Autodesk Inventor part; units mm, degrees
(part 2 of 2)
sketch "スケッチ7" plane through (0, 0, 0) normal (0, 0, 1) x (1, 0, 0)
  line L0 (-15.4359, 10.7396) -> (-13.9558, 2.1157) projected
  line L1 (-1.1431, 4.3146) -> (-2.6232, 12.9386) projected
  line L2 (-2.6232, 12.9386) -> (-15.4359, 10.7396) projected
  line L3 (-8.5367, 11.9237) -> (-3.6088, 12.7694) projected
  line L4 (-14.4503, 10.9088) -> (-9.5223, 11.7545) projected
  line L5 (-15.4359, 10.7396) -> (-13.9558, 2.1157) projected
  line L6 (-2.6232, 12.9386) -> (-15.4359, 10.7396) projected
  line L7 (-1.1431, 4.3146) -> (-2.6232, 12.9386) projected
  line L8 (-8.0423, 3.1306) -> (-12.9702, 2.2848) projected
  line L9 (-13.9558, 2.1157) -> (-1.1431, 4.3146) projected
  line L10 (-13.9558, 2.1157) -> (-1.1431, 4.3146) projected
  line L11 (-7.0686, 4.7383) -> (-2.1618, 5.6993) projected
  line L12 (-1.1804, 5.8915) -> (-7.5593, 4.6422) projected
  line L13 (-7.5593, 4.6422) -> (-1.1804, 5.8915) projected
  line L14 (-9.0295, 11.8391) -> (-7.5495, 3.2152) projected
  line L15 (-7.5495, 3.2152) -> (-9.0295, 11.8391) projected
  line L16 (15.4359, 10.7396) -> (13.9558, 2.1157) projected
  line L17 (1.1431, 4.3146) -> (2.6232, 12.9386) projected
  line L18 (2.6232, 12.9386) -> (15.4359, 10.7396) projected
  line L19 (3.6088, 12.7694) -> (8.5367, 11.9237) projected
  line L20 (9.5223, 11.7545) -> (14.4503, 10.9088) projected
  line L21 (15.4359, 10.7396) -> (13.9558, 2.1157) projected
  line L22 (2.6232, 12.9386) -> (15.4359, 10.7396) projected
  line L23 (1.1431, 4.3146) -> (2.6232, 12.9386) projected
  line L24 (2.1618, 5.6993) -> (7.0686, 4.7383) projected
  line L25 (7.5593, 4.6422) -> (1.1804, 5.8915) projected
  line L26 (1.1804, 5.8915) -> (7.5593, 4.6422) projected
  line L27 (7.5495, 3.2152) -> (9.0295, 11.8391) projected
  line L28 (9.0295, 11.8391) -> (7.5495, 3.2152) projected
  line L29 (13.9558, 2.1157) -> (1.1431, 4.3146) projected
  line L30 (13.9558, 2.1157) -> (1.1431, 4.3146) projected
  line L31 (12.9702, 2.2848) -> (8.0423, 3.1306) projected
  line L32 (-291.6857, -36.6711) -> (324.2647, 69.0399) projected
  line L33 (-324.2647, 69.0399) -> (291.6857, -36.6711) projected
  line L34 (0, 0) -> (0, 10) construction
  line L35 (0, 0) -> (10, 0) construction
  line L36 (0, 0) -> (10, 0) construction
  line L37 (-18, 1.5) -> (-17, 1.5) construction
  line L38 (-18, 11.5) -> (-18, -11.5) construction
  line L39 (-18, -11.5) -> (-20, -11.5) construction
  line L40 (-20, -11.5) -> (-20, 11.5) construction
  line L41 (-28.75, 11.5) -> (-28.75, -11.5) construction
  line L42 (-28.75, -11.5) -> (-20, -11.5) construction
  line L43 (-17, -1.5) -> (-18, -1.5) construction
  line L44 (0, 0) -> (0, 10) construction
  line L45 (17, -20) -> (-17, -20) construction
  line L46 (-20, 11.5) -> (-18, 11.5) construction
  line L47 (-20, 11.5) -> (-28.75, 11.5) construction
  line L48 (-10.5, 21) -> (-14.5, 21) construction
  circle A0 centre (-12.5, 23.5) radius 1 construction
  line L49 (-14.5, 26) -> (-10.5, 21) construction
  line L50 (-10.5, 26) -> (-14.5, 21) construction
  line L51 (-10.5, 26) -> (-10.5, 21) construction
  line L52 (10.5, 26) -> (10.5, 21) construction
  circle A1 centre (12.5, 23.5) radius 1 construction
  line L53 (10.5, 21) -> (14.5, 21) construction
  line L54 (10.5, 26) -> (14.5, 21) construction
  line L55 (10.5, 21) -> (14.5, 26) construction
  circle A2 centre (0, 0) radius 16 construction
  circle A3 centre (0, 0) radius 7.5 construction
  line L56 (20, 11.5) -> (28.75, 11.5) construction
  line L57 (28.75, 11.5) -> (28.75, -11.5) construction
  line L58 (-17, -20) -> (-17, 26) construction
  line L59 (-14.5, 26) -> (-14.5, -20) construction
  line L60 (-17, 26) -> (17, 26) construction
  line L61 (17, -1.5) -> (18, -1.5) construction
  line L62 (18, 1.5) -> (17, 1.5) construction
  line L63 (18, 11.5) -> (18, -11.5) construction
  line L64 (20, 11.5) -> (18, 11.5) construction
  line L65 (18, -11.5) -> (20, -11.5) construction
  line L66 (20, -11.5) -> (20, 11.5) construction
  line L67 (28.75, -11.5) -> (20, -11.5) construction
  line L68 (14.5, 26) -> (14.5, -20) construction
  line L69 (17, 26) -> (17, -20) construction
  line L70 (-14.5, -15) -> (-10.5, -15) construction
  circle A4 centre (-12.5, -17.5) radius 1 construction
  line L71 (-14.5, -15) -> (-10.5, -20) construction
  line L72 (-10.5, -15) -> (-14.5, -20) construction
  line L73 (-10.5, -15) -> (-10.5, -20) construction
  line L74 (10.5, -15) -> (14.5, -15) construction
  circle A5 centre (12.5, -17.5) radius 1 construction
  line L75 (10.5, -20) -> (10.5, -15) construction
  line L76 (14.5, -15) -> (10.5, -20) construction
  line L77 (10.5, -15) -> (14.5, -20) construction
  line L78 (29.25, -41.1836) -> (-29.25, -41.1836) construction
  line L79 (-29.25, -41.1836) -> (29.25, -41.1836) projected
  line L80 (0, 0) -> (0, 10) construction
  line L81 (0, 0) -> (0, 10) construction
  line L82 (20, 11.5) -> (18, 11.5) construction
  line L83 (2.6232, 12.9386) -> (1.1431, 4.3146) construction
  line L84 (9.0295, 11.8391) -> (2.6232, 12.9386) construction
  line L85 (8.4099, 11.1845) -> (3.4819, 12.0302) construction
  line L86 (3.4819, 12.0302) -> (2.6362, 7.1023) construction
  line L87 (8.4099, 11.1845) -> (2.6362, 7.1023) construction
  line L88 (7.5641, 6.2565) -> (3.4819, 12.0302) construction
  line L89 (2.6362, 7.1023) -> (7.5641, 6.2565) construction
  line L90 (7.9301, 5.4327) -> (1.5237, 6.5322) construction
  line L91 (7.5641, 6.2565) -> (8.4099, 11.1845) construction
  line L92 (13.4777, 5.2416) -> (14.3234, 10.1696) construction
  line L93 (17, 8.5) -> (17, -8.5) construction
  line L94 (7.5495, 3.2152) -> (9.0295, 11.8391) construction
  line L95 (9.3955, 11.0153) -> (8.5497, 6.0874) construction
  line L96 (8.5497, 6.0874) -> (13.4777, 5.2416) construction
  line L97 (13.4777, 5.2416) -> (9.3955, 11.0153) construction
  line L98 (13.9005, 7.7056) -> (8.9726, 8.5513) construction
  line L99 (14.3234, 10.1696) -> (9.3955, 11.0153) construction
  line L100 (15.4359, 10.7396) -> (9.0295, 11.8391) construction
  line L101 (14.1851, 3.4517) -> (7.8081, 4.722) construction
  line L102 (10.5062, 2.7077) -> (11.0137, 5.6645) construction
  line L103 (13.9558, 2.1157) -> (15.4359, 10.7396) construction
  line L104 (7.5495, 3.2152) -> (13.9558, 2.1157) construction
  line L105 (9.0295, 11.8391) -> (7.5495, 3.2152) construction
  circle A6 centre (0, 0) radius 4.25 construction
  line L106 (1.1431, 4.3146) -> (7.5495, 3.2152) construction
  line L107 (29.25, 8.5) -> (17, 8.5) construction
  line L108 (-2.6232, 12.9386) -> (-1.1431, 4.3146) construction
  line L109 (-3.4819, 12.0302) -> (-2.6362, 7.1023) construction
  line L110 (-8.4099, 11.1845) -> (-3.4819, 12.0302) construction
  line L111 (-7.5641, 6.2565) -> (-3.4819, 12.0302) construction
  line L112 (-8.4099, 11.1845) -> (-2.6362, 7.1023) construction
  line L113 (-7.987, 8.7205) -> (-3.059, 9.5662) construction
  line L114 (-4.5927, 3.7226) -> (-5.1001, 6.6794) construction
  line L115 (-2.6362, 7.1023) -> (-7.5641, 6.2565) construction
  line L116 (-7.9301, 5.4327) -> (-1.5237, 6.5322) construction
  line L117 (-1.1431, 4.3146) -> (-7.5495, 3.2152) construction
  line L118 (-13.4777, 5.2416) -> (-9.3955, 11.0153) construction
  line L119 (-10.5062, 2.7077) -> (-11.0137, 5.6645) construction
  line L120 (-8.5497, 6.0874) -> (-13.4777, 5.2416) construction
  circle A7 centre (12.5, -17.5) radius 1 construction
  line L121 (14.5, -15) -> (10.5, -20) construction
  line L122 (10.3558, 32.528) -> (9.7395, 39.5722) construction
  line L123 (10.2875, 31.2799) -> (5.3082, 35.458) construction
  line L124 (10.3558, 32.528) -> (6.5255, 35.7419) construction
  line L125 (6.5255, 35.7419) -> (9.7395, 39.5722) construction
  line L126 (13.5697, 36.3582) -> (10.3558, 32.528) construction
  line L127 (6.5255, 35.7419) -> (13.5697, 36.3582) construction
  circle A8 centre (6.8337, 32.2199) radius 0.625 construction
  circle A9 centre (6.8337, 32.2199) radius 0.8 projected
  line L128 (9.7395, 39.5722) -> (13.5697, 36.3582) construction
  line L129 (5.3082, 35.458) -> (14.787, 36.6422) construction
  line L130 (14.787, 36.6422) -> (10.2875, 31.2799) construction
  circle A10 centre (13.6863, 32.9968) radius 1.5 construction
  circle A11 centre (13.6863, 32.9968) radius 0.8 projected
  line L131 (-17, 8.5) -> (-17, -8.5) construction
  line L132 (-7.5641, 6.2565) -> (-8.4099, 11.1845) construction
  line L133 (-7.5495, 3.2152) -> (-9.0295, 11.8391) construction
  line L134 (-14.3364, 4.3333) -> (-7.9301, 5.4327) construction
  line L135 (-7.5495, 3.2152) -> (-13.9558, 2.1157) construction
  line L136 (-13.4777, 5.2416) -> (-14.3234, 10.1696) construction
  line L137 (-15.4359, 10.7396) -> (-13.9558, 2.1157) construction
  line L138 (-13.9558, 2.1157) -> (-15.4359, 10.7396) construction
  line L139 (-14.3234, 10.1696) -> (-8.5497, 6.0874) construction
  line L140 (-13.9005, 7.7056) -> (-8.9726, 8.5513) construction
  line L141 (-14.3234, 10.1696) -> (-9.3955, 11.0153) construction
  line L142 (-15.4359, 10.7396) -> (-9.0295, 11.8391) construction
  line L143 (-9.7365, 26) -> (-17, 26) projected
  line L144 (-20, 11.5) -> (-18, 11.5) construction
  line L145 (-18, -11.5) -> (-20, -11.5) construction
  line L146 (-18, 11.5) -> (-18, -11.5) construction
  line L147 (-20, -11.5) -> (-20, 11.5) construction
  line L148 (-10.5, 26) -> (-10.5, 21) construction
  line L149 (-10.5, 21) -> (-14.5, 21) construction
  circle A12 centre (-6.8337, 32.2199) radius 0.625 construction
  circle A13 centre (-6.8337, 32.2199) radius 0.8 construction
  circle A14 centre (-6.8337, 32.2199) radius 1.5 construction
  line L150 (-5.3082, 35.458) -> (-10.2875, 31.2799) construction
  line L151 (-6.5255, 35.7419) -> (-10.3558, 32.528) construction
  line L152 (-13.5697, 36.3582) -> (-6.5255, 35.7419) construction
  line L153 (-10.0476, 36.0501) -> (-6.8337, 32.2199) construction
  line L154 (3.695, 18.0905) -> (-3.695, 18.0905) projected
  line L155 (-9.7365, 22.9366) -> (-3.695, 18.0905) projected
  circle A15 centre (-12.5, 23.5) radius 1 construction
  line L156 (-14.5, 26) -> (-10.5, 21) construction
  line L157 (-10.5, 26) -> (-14.5, 21) construction
  line L158 (-5.3082, 35.458) -> (-14.787, 36.6422) construction
  line L159 (-29.25, 8.5) -> (-17, 8.5) construction
  line L160 (-28.75, -11.5) -> (-20, -11.5) construction
  line L161 (-28.75, 11.5) -> (-28.75, -11.5) construction
  line L162 (-20, 11.5) -> (-28.75, 11.5) construction
  line L163 (-25.25, 15.774) -> (-13.111, 37.7059) projected
  line L164 (-6.6466, -20.8804) -> (-17, -20.8804) projected
  line L165 (-17, -20.8804) -> (-17, -14.5) projected
  line L166 (-25.25, -19.2406) -> (-7.307, -37.1836) projected
  line L167 (-29.25, -20.8975) -> (-8.9639, -41.1836) projected
  line L168 (-17, -14.5) -> (-25.25, -14.5) projected
  line L169 (-25.25, -14.5) -> (-25.25, -19.2406) projected
  line L170 (-7.307, -37.1836) -> (7.307, -37.1836) projected
  line L171 (-9.7395, 39.5722) -> (-6.5255, 35.7419) construction
  line L172 (-9.8077, 40.8203) -> (-5.3082, 35.458) construction
  circle A16 centre (6.8337, 32.2199) radius 1.5 construction
  line L173 (-13.111, 37.7059) -> (13.111, 37.7059) projected
  line L174 (-29.25, 41.8164) -> (29.25, 41.8164) projected
  line L175 (5.3082, 35.458) -> (9.8077, 40.8203) construction
  line L176 (9.8077, 40.8203) -> (10.2875, 31.2799) construction
  line L177 (10.2875, 31.2799) -> (12.5856, 29.3515) construction
  line L178 (9.8077, 40.8203) -> (14.787, 36.6422) construction
  line L179 (17.0851, 34.7138) -> (14.787, 36.6422) construction
  line L180 (12.5856, 29.3515) -> (17.0851, 34.7138) construction
  line L181 (-14.787, 36.6422) -> (-9.8077, 40.8203) construction
  line L182 (-13.5697, 36.3582) -> (-9.7395, 39.5722) construction
  line L183 (-14.787, 36.6422) -> (-17.0851, 34.7138) construction
  line L184 (-9.7395, 39.5722) -> (-10.3558, 32.528) construction
  line L185 (-10.3558, 32.528) -> (-13.5697, 36.3582) construction
  line L186 (-9.8077, 40.8203) -> (-10.2875, 31.2799) construction
  line L187 (-10.2875, 31.2799) -> (-14.787, 36.6422) construction
  line L188 (-17.0851, 34.7138) -> (-12.5856, 29.3515) construction
  line L189 (-12.5856, 29.3515) -> (-10.2875, 31.2799) construction
  line L190 (-9.7365, 22.9366) -> (-9.7365, 26) projected
  circle A17 centre (-13.6863, 32.9968) radius 0.625 construction
  circle A18 centre (-13.6863, 32.9968) radius 0.8 construction
  circle A19 centre (-13.6863, 32.9968) radius 1.5 construction
  line L191 (4.5158, -27.0126) -> (-4.5158, -27.0126) projected
  line L192 (29.25, -20.8975) -> (8.9639, -41.1836) projected
  line L193 (6.6466, -20.8804) -> (4.5158, -27.0126) projected
  line L194 (17, -20.8804) -> (6.6466, -20.8804) projected
  line L195 (7.307, -37.1836) -> (25.25, -19.2406) projected
  line L196 (-10.5, -15) -> (-10.5, -20) construction
  line L197 (10.5, -20) -> (10.5, -15) construction
  line L198 (10.5, -15) -> (14.5, -15) construction
  line L199 (10.5, -15) -> (14.5, -20) construction
  line L200 (17, -14.5) -> (17, -20.8804) projected
  line L201 (25.25, -14.5) -> (17, -14.5) projected
  line L202 (28.75, -11.5) -> (20, -11.5) construction
  line L203 (-17, -8.5) -> (-29.25, -8.5) construction
  line L204 (-17, -1.5) -> (-18, -1.5) construction
  line L205 (0, 0) -> (10, 0) construction
  line L206 (-18, 1.5) -> (-17, 1.5) construction
  line L207 (-29.25, -41.1836) -> (-29.25, 41.8164) construction
  line L208 (29.25, 41.8164) -> (29.25, -41.1836) construction
  line L209 (20, 11.5) -> (28.75, 11.5) construction
  line L210 (28.75, 11.5) -> (28.75, -11.5) construction
  line L211 (17, 26) -> (17, -20) construction
  line L212 (14.5, 26) -> (14.5, -20) construction
  line L213 (-4.5158, -27.0126) -> (-6.6466, -20.8804) projected
  line L214 (0, 0) -> (10, 0) construction
  circle A20 centre (0, 0) radius 7.5 construction
  circle A21 centre (0, 0) radius 16 construction
  line L215 (-14.5, 26) -> (-14.5, -20) construction
  line L216 (-9.0295, 11.8391) -> (-2.6232, 12.9386) construction
  line L217 (-14.5, -15) -> (-10.5, -15) construction
  circle A22 centre (-12.5, -17.5) radius 1 construction
  line L218 (17, -20) -> (-17, -20) construction
  line L219 (-17, -20) -> (-17, 26) construction
  line L220 (-10.5, -15) -> (-14.5, -20) construction
  line L221 (-14.5, -15) -> (-10.5, -20) construction
  line L222 (10.5, 21) -> (14.5, 21) construction
  circle A23 centre (12.5, 23.5) radius 1 construction
  line L223 (10.5, 26) -> (14.5, 21) construction
  line L224 (10.5, 21) -> (14.5, 26) construction
  line L225 (10.5, 26) -> (10.5, 21) construction
  line L226 (9.7365, 22.9366) -> (3.695, 18.0905) projected
  line L227 (9.7365, 22.9366) -> (9.7365, 26) projected
  circle A24 centre (13.6863, 32.9968) radius 0.625 construction
  line L228 (9.7365, 26) -> (17, 26) projected
  line L229 (17, 26) -> (17, 14.5) projected
  line L230 (13.111, 37.7059) -> (25.25, 15.774) projected
  line L231 (29.25, 15.7886) -> (14.2228, 41.8164) projected
  line L232 (25.25, 15.774) -> (25.25, 14.5) projected
  line L233 (25.25, 14.5) -> (17, 14.5) projected
  line L234 (17, -1.5) -> (18, -1.5) construction
  line L235 (18, -11.5) -> (20, -11.5) construction
  line L236 (18, 11.5) -> (18, -11.5) construction
  line L237 (17, -8.5) -> (29.25, -8.5) construction
  line L238 (20, -11.5) -> (20, 11.5) construction
  line L239 (-17, 26) -> (17, 26) construction
  line L240 (-25.25, 14.5) -> (-25.25, 15.774) projected
  line L241 (-17, 14.5) -> (-25.25, 14.5) projected
  line L242 (-17, 26) -> (-17, 14.5) projected
  line L243 (-29.25, 15.7886) -> (-14.2228, 41.8164) projected
  line L244 (-9.3955, 11.0153) -> (-8.5497, 6.0874) construction
  line L245 (-9.0295, 11.8391) -> (-7.5495, 3.2152) construction
  line L246 (14.3234, 10.1696) -> (8.5497, 6.0874) construction
  line L247 (18, 1.5) -> (17, 1.5) construction
  line L248 (25.25, -19.2406) -> (25.25, -14.5) projected
  line L249 (0, 0) -> (0, 10) construction
  line L250 (0, 0) -> (0, 10) construction
  line L251 (-2.6362, 7.1023) -> (-7.5641, 6.2565) construction
  line L252 (-7.987, 8.7205) -> (-3.059, 9.5662) construction
  line L253 (-8.4099, 11.1845) -> (-2.6362, 7.1023) construction
  line L254 (-7.5641, 6.2565) -> (-3.4819, 12.0302) construction
  line L255 (0, 0) -> (10, 0) construction
  line L256 (0, 0) -> (10, 0) construction
  circle A25 centre (0, 0) radius 7.5 construction
  line L257 (-18, 11.5) -> (-18, -11.5) construction
  line L258 (-18, 11.5) -> (-18, -11.5) construction
  line L259 (-14.5, -15) -> (-10.5, -15) construction
  line L260 (10.5, -15) -> (14.5, -15) construction
  line L261 (10.5, -20) -> (10.5, -15) construction
  line L262 (10.5, -15) -> (14.5, -20) construction
  line L263 (17, -20) -> (-17, -20) construction
  line L264 (17, -20) -> (-17, -20) construction
  circle A26 centre (0, 0) radius 16 construction
  circle A27 centre (0, 0) radius 16 construction
  line L265 (-10.5, -15) -> (-10.5, -20) construction
  line L266 (-10.5, -15) -> (-14.5, -20) construction
  line L267 (-14.5, 26) -> (-14.5, -20) construction
  line L268 (-14.5, 26) -> (-14.5, -20) construction
  line L269 (-17, -20) -> (-17, 26) construction
  line L270 (-17, -20) -> (-17, 26) construction
  line L271 (-10.5, 21) -> (-14.5, 21) construction
  line L272 (-7.5641, 6.2565) -> (-8.4099, 11.1845) construction
  line L273 (-17, -1.5) -> (-18, -1.5) construction
  line L274 (-10.5, 26) -> (-14.5, 21) construction
  line L275 (-14.5, 26) -> (-10.5, 21) construction
  line L276 (-10.5, 21) -> (-14.5, 21) construction
  line L277 (-10.5, 26) -> (-10.5, 21) construction
  line L278 (10.5, 21) -> (14.5, 21) construction
  line L279 (10.5, 26) -> (14.5, 21) construction
  line L280 (-9.0295, 11.8391) -> (-2.6232, 12.9386) projected
  line L281 (-18, -11.5) -> (-20, -11.5) construction
  line L282 (-18, -11.5) -> (-20, -11.5) construction
  line L283 (-18, 1.5) -> (-17, 1.5) construction
  line L284 (-18, 1.5) -> (-17, 1.5) construction
  circle A28 centre (-12.5, 23.5) radius 1 construction
  line L285 (10.5, 26) -> (10.5, 21) construction
  circle A29 centre (12.5, 23.5) radius 1 construction
  circle A30 centre (-12.5, 23.5) radius 1 construction
  line L286 (-14.5, 26) -> (-10.5, 21) construction
  line L287 (-10.5, 26) -> (-14.5, 21) construction
  circle A31 centre (-13.6863, 32.9968) radius 1.5 construction
  line L288 (-17.0851, 34.7138) -> (-12.5856, 29.3515) construction
  circle A32 centre (-6.8337, 32.2199) radius 1.5 construction
  line L289 (-10.2875, 31.2799) -> (-14.787, 36.6422) construction
  line L290 (-5.3082, 35.458) -> (-14.787, 36.6422) construction
  line L291 (-13.5697, 36.3582) -> (-9.7395, 39.5722) construction
  line L292 (-14.787, 36.6422) -> (-9.8077, 40.8203) construction
  line L293 (10.5, 21) -> (14.5, 26) construction
  line L294 (12.5856, 29.3515) -> (17.0851, 34.7138) construction
  line L295 (-14.787, 36.6422) -> (-17.0851, 34.7138) construction
  circle A33 centre (12.5, -17.5) radius 1 construction
  line L296 (14.5, -15) -> (10.5, -20) construction
  circle A34 centre (-12.5, -17.5) radius 1 construction
  line L297 (-14.5, -15) -> (-10.5, -20) construction
  circle A35 centre (-12.5, -17.5) radius 1 construction
  line L298 (-14.5, -15) -> (-10.5, -20) construction
  line L299 (-10.5, 26) -> (-10.5, 21) construction
  line L300 (-15.4359, 10.7396) -> (-9.0295, 11.8391) projected
  line L301 (-14.3364, 4.3333) -> (-7.9301, 5.4327) projected
  line L302 (-13.9558, 2.1157) -> (-15.4359, 10.7396) projected
  line L303 (-7.5495, 3.2152) -> (-13.9558, 2.1157) projected
  line L304 (-2.6232, 12.9386) -> (-1.1431, 4.3146) projected
  line L305 (0, 0) -> (0, 10) construction
  line L306 (0, 0) -> (0, 10) construction
  line L307 (-4.5927, 3.7226) -> (-5.1001, 6.6794) construction
  circle A36 centre (0, 0) radius 7.5 construction
  line L308 (0, 0) -> (10, 0) construction
  line L309 (0, 0) -> (10, 0) construction
  line L310 (10.3558, 32.528) -> (9.7395, 39.5722) construction
  line L311 (-20, 11.5) -> (-18, 11.5) construction
  line L312 (-20, 11.5) -> (-18, 11.5) construction
  line L313 (-20, -11.5) -> (-20, 11.5) construction
  line L314 (-20, 11.5) -> (-28.75, 11.5) construction
  line L315 (-28.75, 11.5) -> (-28.75, -11.5) construction
  line L316 (-28.75, -11.5) -> (-20, -11.5) construction
  line L317 (-7.9301, 5.4327) -> (-1.5237, 6.5322) projected
  line L318 (-1.1431, 4.3146) -> (-7.5495, 3.2152) projected
  line L319 (-7.5495, 3.2152) -> (-9.0295, 11.8391) projected
  line L320 (10.5, -15) -> (14.5, -15) construction
  line L321 (-20, 11.5) -> (-28.75, 11.5) construction
  line L322 (-17, -1.5) -> (-18, -1.5) construction
  line L323 (-29.25, 8.5) -> (-17, 8.5) construction
  line L324 (-28.75, 11.5) -> (-28.75, -11.5) construction
  line L325 (-28.75, -11.5) -> (-20, -11.5) construction
  line L326 (-20, -11.5) -> (-20, 11.5) construction
  line L327 (18, 11.5) -> (18, -11.5) construction
  line L328 (20, -11.5) -> (20, 11.5) construction
  line L329 (17, -1.5) -> (18, -1.5) construction
  line L330 (18, 1.5) -> (17, 1.5) construction
  line L331 (20, 11.5) -> (18, 11.5) construction
  line L332 (18, -11.5) -> (20, -11.5) construction
  line L333 (17.0851, 34.7138) -> (14.787, 36.6422) construction
  line L334 (13.5697, 36.3582) -> (10.3558, 32.528) construction
  line L335 (14.787, 36.6422) -> (10.2875, 31.2799) construction
  line L336 (10.5, 21) -> (14.5, 21) construction
  circle A37 centre (12.5, 23.5) radius 1 construction
  line L337 (10.5, 26) -> (14.5, 21) construction
  line L338 (10.5, 26) -> (10.5, 21) construction
  line L339 (10.5, 21) -> (14.5, 26) construction
  circle A38 centre (13.6863, 32.9968) radius 0.625 construction
  circle A39 centre (13.6863, 32.9968) radius 1.5 construction
  line L340 (9.8077, 40.8203) -> (14.787, 36.6422) construction
  line L341 (20, -11.5) -> (20, 11.5) construction
  line L342 (9.8077, 40.8203) -> (10.2875, 31.2799) construction
  line L343 (20, 11.5) -> (18, 11.5) construction
  line L344 (18, 1.5) -> (17, 1.5) construction
  line L345 (17, -1.5) -> (18, -1.5) construction
  line L346 (18, -11.5) -> (20, -11.5) construction
  line L347 (18, 11.5) -> (18, -11.5) construction
  line L348 (-17, 8.5) -> (-17, -8.5) construction
  line L349 (10.5, -20) -> (10.5, -15) construction
  line L350 (-17, -8.5) -> (-29.25, -8.5) construction
  line L351 (-10.5, -15) -> (-10.5, -20) construction
  line L352 (14.5, 26) -> (14.5, -20) construction
  line L353 (17, 26) -> (17, -20) construction
  line L354 (20, 11.5) -> (28.75, 11.5) construction
  line L355 (28.75, 11.5) -> (28.75, -11.5) construction
  line L356 (28.75, -11.5) -> (20, -11.5) construction
  line L357 (-8.4099, 11.1845) -> (-3.4819, 12.0302) construction
  line L358 (-3.4819, 12.0302) -> (-2.6362, 7.1023) construction
  line L359 (17, 8.5) -> (17, -8.5) construction
  line L360 (14.5, 26) -> (14.5, -20) construction
  line L361 (17, 26) -> (17, -20) construction
  line L362 (28.75, 11.5) -> (28.75, -11.5) construction
  line L363 (28.75, -11.5) -> (20, -11.5) construction
  circle A40 centre (12.5, -17.5) radius 1 construction
  line L364 (10.5, -15) -> (14.5, -20) construction
  line L365 (14.5, -15) -> (10.5, -20) construction
  line L366 (-14.5, -15) -> (-10.5, -15) construction
  line L367 (-10.5, -15) -> (-14.5, -20) construction
  line L368 (29.25, 8.5) -> (17, 8.5) construction
  line L369 (17, -8.5) -> (29.25, -8.5) construction
  line L370 (20, 11.5) -> (28.75, 11.5) construction
  line L371 (6.5255, 35.7419) -> (9.7395, 39.5722) construction
  line L372 (29.25, -41.1836) -> (-29.25, -41.1836) construction
  line L373 (5.3082, 35.458) -> (9.8077, 40.8203) construction
  line L374 (9.7395, 39.5722) -> (13.5697, 36.3582) construction
  line L375 (-9.7395, 39.5722) -> (-6.5255, 35.7419) construction
  line L376 (-9.8077, 40.8203) -> (-5.3082, 35.458) construction
  line L377 (-6.5255, 35.7419) -> (-10.3558, 32.528) construction
  line L378 (-5.3082, 35.458) -> (-10.2875, 31.2799) construction
  circle A41 centre (-6.8337, 32.2199) radius 0.625 construction
  line L379 (-9.7395, 39.5722) -> (-10.3558, 32.528) construction
  line L380 (-9.8077, 40.8203) -> (-10.2875, 31.2799) construction
  line L381 (-29.25, -41.1836) -> (-29.25, 41.8164) construction
  circle A42 centre (13.6863, 32.9968) radius 0.8 projected
  line L382 (6.5255, 35.7419) -> (13.5697, 36.3582) construction
  circle A43 centre (-13.6863, 32.9968) radius 0.625 construction
  circle A44 centre (-13.6863, 32.9968) radius 0.8 construction
  circle A45 centre (-6.8337, 32.2199) radius 0.8 construction
  line L383 (-10.3558, 32.528) -> (-13.5697, 36.3582) construction
  line L384 (-13.5697, 36.3582) -> (-6.5255, 35.7419) construction
  circle A46 centre (6.8337, 32.2199) radius 0.625 construction
  line L385 (10.2875, 31.2799) -> (5.3082, 35.458) construction
  line L386 (10.3558, 32.528) -> (6.5255, 35.7419) construction
  line L387 (5.3082, 35.458) -> (14.787, 36.6422) construction
  circle A47 centre (6.8337, 32.2199) radius 0.8 projected
  line L388 (-15.4359, 10.7396) -> (-20.1374, 14.5)
  line L389 (-17, 15.7784) -> (-14.1003, 10.9688)
  point P0 (-12.5, -17.5)
  point P1 (1.5237, 6.5322)
  point P2 (-5.523, 9.1434)
  point P3 (-5.523, 9.1434)
  point P4 (-5.523, 9.1434)
  point P5 (-1.5237, 6.5322)
  point P6 (-11.4366, 8.1285)
  point P7 (-11.4366, 8.1285)
  point P8 (10.0476, 36.0501)
  point P9 (-10.0476, 36.0501)
  point P10 (25.25, 25.1515)
  point P11 (11.4366, 8.1285)
  point P12 (11.4366, 8.1285)
  point P13 (-1.5237, 6.5322)
  point P14 (-10.0476, 36.0501)
  point P15 (-5.523, 9.1434)
  point P16 (10.0476, 36.0501)
  point P17 (-12.5, -17.5)
  point P18 (-14.1003, 10.9688)
  constraints: 4 end point, 2 point on line, 124 other
extrude "押し出し10" add sketch "スケッチ7" along normal blind 1 contours L388 L241 L242 L389 L2
extrude "押し出し11" cut sketch "スケッチ4" along normal blind 10 contours L168 L166 L167 L169
mirror "ミラー4" about plane through (0, 0, 0) normal (1, 0, 0) of "押し出し11"
ref_plane "作業平面4" through (15.4359, 10.7396, 7) normal (-0.1691495, -0.9855904, 0) x (-0.9855904, 0.1691495, 0)
